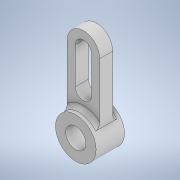
# Autodesk Inventor part: 13
Saved by Autodesk Inventor 2022 (Build 260153000, 153)
## iProperties
Created: 2022-03-14
Part Number: 13
Material: Všeobecné
Document SubType Name: Modeling
Designer: Šimon
Density: 1 g/cm^3
Appearance: Výchozí
Author: Šimon
Autodesk Inventor part; units mm, degrees
ref_plane "YZ Plane" through (0, 0, 0) normal (1, 0, 0) x (0, 1, 0)
ref_plane "XZ Plane" through (0, 0, 0) normal (0, 1, 0) x (-1, 0, 0)
ref_plane "XY Plane" through (0, 0, 0) normal (0, 0, 1) x (1, 0, 0)
sketch "Náčrt1" plane through (0, 0, 0) normal (0, 0, 1) x (1, 0, 0)
  circle A0 centre (0, 0) radius 25
  dimension "d0" = 50
  constraints: 1 centre point, 1 coincident
  measures "d0" diameter of A0
extrude "Vysunutí1" add sketch "Náčrt1" against normal blind 25.5
sketch "Náčrt2" plane through (0, 0, 0) normal (0, 0, 1) x (1, 0, 0)
  circle A0 centre (0, 0) radius 12.5
  dimension "d3" = 25
  constraints: 1 centre point, 1 coincident
  measures "d3" diameter of A0
extrude "Vysunutí2" cut sketch "Náčrt2" against normal blind 35
sketch "Náčrt3" plane through (0, 0, 0) normal (0, 0, 1) x (1, 0, 0)
  circle A0 centre (0, 0) radius 25 projected
  line L0 (20, 15) -> (20, 90)
  arc A1 (20, 90) -> (-20, 90) centre (0, 90) ccw
  line L1 (-20, 90) -> (-20, 15)
  arc A2 (10, 90) -> (-10, 90) centre (0, 90) ccw
  line L2 (-10, 90) -> (-10, 45)
  arc A3 (-10, 45) -> (10, 45) centre (0, 45) ccw
  line L3 (10, 45) -> (10, 90)
  arc A4 (20, 15) -> (-20, 15) centre (0, 0) ccw
  dimension "d7" = 90
  dimension "d8" = 40
  dimension "d9" = 20
  dimension "d10" = 20
  dimension "d11" = 10
  dimension "d12" = 45
  constraints: 10 point on circle, 8 end point, 4 centre point, 2 parallel, 2 tangent, 1 coincident, 1 concentric, 1 vertical
  measures "d7" vertical distance of A0.centre L0.end
  measures "d8" distance of L0.end L1.start
  measures "d9" radius of A1
  measures "d10" distance of L2.start A2.start
  measures "d11" radius of A2
  measures "d12" distance of L2.start L2.end
extrude "Vysunutí3" add sketch "Náčrt3" against normal blind 16 contours A0 L1 A1 L0
sketch "Náčrt4" plane through (0, 0, 0) normal (0, 0, 1) x (1, 0, 0)
  circle A0 centre (0, 0) radius 25
  circle A1 centre (0, 0) radius 25 projected
  circle A2 centre (0, 0) radius 12.5
  constraints: 2 centre point, 2 coincident
extrude "Vysunutí4" add sketch "Náčrt4" along normal blind 9.5
fillet "Zaoblení1" radius 5 1 edges at (0, 25, 0)
fillet "Zaoblení2" radius 5 1 edges at (0, 25, -16)
